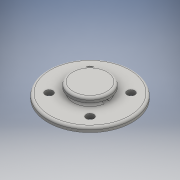
# Autodesk Inventor part: pulley
Saved by Autodesk Inventor 2016 (Build 200138000, 138)
## iProperties
Created: 2016-08-24
Part Number: pulley
Material: Generic
Document SubType Name: Modeling
Designer: Hamid Osooli
Density: 1 g/cm^3
Appearance: Default
Author: Hamid Osooli
Autodesk Inventor part; units mm, degrees
ref_plane "YZ Plane" through (0, 0, 0) normal (1, 0, 0) x (0, 1, 0)
ref_plane "XZ Plane" through (0, 0, 0) normal (0, 1, 0) x (-1, 0, 0)
ref_plane "XY Plane" through (0, 0, 0) normal (0, 0, 1) x (1, 0, 0)
sketch "Sketch1" plane through (0, 0, 0) normal (0, 0, 1) x (1, 0, 0)
  circle A0 centre (0, 0) radius 8.7
  dimension "d0" = 17.4
  constraints: 1 centre point, 1 coincident
  measures "d0" diameter of A0
extrude "Extrusion1" add sketch "Sketch1" along normal blind 1
sketch "Sketch2" plane through (0, 0, 1) normal (0, 0, 1) x (1, 0, 0)
  circle A0 centre (4.2426, 4.2426) radius 0.8
  circle A1 centre (-4.2426, 4.2426) radius 0.8
  circle A2 centre (-4.2426, -4.2426) radius 0.8
  circle A3 centre (4.2426, -4.2426) radius 0.8
  dimension "d9" = 1.6
  dimension "d10" = 1.6
  dimension "d11" = 1.6
  dimension "d12" = 1.6
  constraints: 4 centre point
  measures "d9" diameter of A0
  measures "d10" diameter of A1
  measures "d11" diameter of A2
  measures "d12" diameter of A3
extrude "Extrusion2" cut sketch "Sketch2" against normal up to next
sketch "Sketch3" plane through (0, 0, 0) normal (0, 0, -1) x (-1, 0, 0)
  circle A0 centre (0, 0) radius 2.8
  dimension "d15" = 5.6
  constraints: 1 centre point, 1 coincident
  measures "d15" diameter of A0
extrude "Extrusion3" cut sketch "Sketch3" against normal blind 0.5
fillet "Fillet1" radius 0.5 1 edges at (2.8, 0, 0.5)
fillet "Fillet4" radius 0.5 1 edges at (-8.7, 0, 1)
sketch "Sketch7" plane through (0, 0, 1) normal (0, 0, 1) x (1, 0, 0)
  line L0 (-2.958, 0.5) -> (2.958, 0.5)
  line L1 (2.958, -0.5) -> (-2.958, -0.5)
  arc A0 (2.958, 0.5) -> (-2.958, 0.5) centre (0, 0) ccw
  arc A1 (-2.958, -0.5) -> (2.958, -0.5) centre (0, 0) ccw
  point P0 (0, 0)
  constraints: 4 end point, 4 point on circle, 2 centre point
extrude "Extrusion7" add sketch "Sketch7" along normal blind 1
sketch "Sketch8" plane through (0, 0, 2) normal (0, 0, 1) x (1, 0, 0)
  circle A0 centre (0, 0) radius 4
  dimension "d38" = 8
  constraints: 1 centre point, 1 coincident
  measures "d38" diameter of A0
extrude "Extrusion8" add sketch "Sketch8" along normal blind 1
fillet "Fillet5" radius 0.5 4 edges at (0, -3, 2) (0, 3, 2) (0, 3, 1) (0, -3, 1)
fillet "Fillet6" radius 0.5 1 edges at (-4, 0, 3)
body "Solid1"
